Autodesk Fusion 360 part; units mm, degrees
note: some values were not read from the file. Set by a fixed rule: which sketch regions a step uses.
(part 2 of 2)
  spline S320 degree 3 poles (36.333, 6.3383) (36.524, 6.2477) (36.7934, 6.1802) (37.1049, 6.2117) knots 0 0 0 0 1 1 1 1
  spline S321 degree 3 poles (37.1049, 6.2117) (37.645, 6.2677) (38.0601, 6.5293) (38.0394, 7.1055) knots 0 0 0 0 1 1 1 1
  line L71 (38.0394, 7.1055) -> (37.6236, 7.1055)
  spline S322 degree 3 poles (37.6236, 7.1055) (37.6105, 6.9605) (37.5622, 6.7963) (37.4701, 6.7127) knots 0 0 0 0 1 1 1 1
  spline S323 degree 3 poles (37.4701, 6.7127) (37.2798, 6.5385) (36.9031, 6.5393) (36.613, 6.639) knots 0 0 0 0 1 1 1 1
  spline S324 degree 3 poles (36.613, 6.639) (36.3852, 6.7173) (36.3092, 7.0603) (36.399, 7.2368) knots 0 0 0 0 1 1 1 1
  spline S325 degree 3 poles (36.399, 7.2368) (36.4964, 7.427) (36.9998, 7.3472) (37.4548, 7.4539) knots 0 0 0 0 1 1 1 1
  spline S326 degree 3 poles (37.4548, 7.4539) (37.7601, 7.5268) (38.0279, 7.6626) (38.1292, 8.0232) knots 0 0 0 0 1 1 1 1
  spline S327 degree 3 poles (38.1292, 8.0232) (38.196, 8.255) (38.1737, 8.5534) (38.0617, 8.7291) knots 0 0 0 0 1 1 1 1
  spline S328 degree 3 poles (38.0617, 8.7291) (37.797, 9.1389) (37.0911, 9.1757) (36.6506, 8.9002) knots 0 0 0 0 1 1 1 1
  spline S329 degree 3 poles (36.6506, 8.9002) (36.5463, 8.8343) (36.4488, 8.7314) (36.3591, 8.6493) knots 0 0 0 0 1 1 1 1
  spline S330 degree 3 poles (36.3591, 8.6493) (36.3399, 9.0276) (36.0429, 9.1289) (35.6248, 9.0023) knots 0 0 0 0 1 1 1 1
  line L72 (35.6248, 9.0023) -> (35.6271, 8.6678)
  spline S331 degree 3 poles (35.6271, 8.6678) (35.7475, 8.7023) (35.9348, 8.7222) (35.9348, 8.5573) knots 0 0 0 0 1 1 1 1
  spline S332 degree 3 poles (36.4465, 8.3186) (36.5708, 8.5642) (36.9269, 8.7115) (37.2399, 8.7115) knots 0 0 0 0 1 1 1 1
  spline S333 degree 3 poles (37.2399, 8.7115) (37.4655, 8.7115) (37.6619, 8.6079) (37.7003, 8.3301) knots 0 0 0 0 1 1 1 1
  spline S334 degree 3 poles (37.7003, 8.3301) (37.7225, 8.2166) (37.7011, 8.0984) (37.6412, 7.9994) knots 0 0 0 0 1 1 1 1
  spline S335 degree 3 poles (37.6412, 7.9994) (37.5507, 7.859) (37.3404, 7.7961) (36.9921, 7.7639) knots 0 0 0 0 1 1 1 1
  spline S336 degree 3 poles (36.9921, 7.7639) (36.7642, 7.7439) (36.4887, 7.6779) (36.3782, 7.6173) knots 0 0 0 0 1 1 1 1
  spline S337 degree 3 poles (36.3782, 7.6173) (36.3744, 7.8414) (36.366, 8.1629) (36.4458, 8.3179) knots 0 0 0 0 1 1 1 1
  line L73 (36.4458, 8.3179) -> (36.4465, 8.3186)
  line L74 (32.4735, 5.2733) -> (32.0277, 5.2733)
  line L75 (32.0277, 5.2733) -> (32.0277, 9.0138)
  line L76 (32.0277, 9.0138) -> (32.4735, 9.0138)
  line L77 (32.4735, 9.0138) -> (32.4735, 5.2733)
extrude "Extrude3" add sketch "Sketch3" along normal blind 0.0254 separate body contours S0 L0 S1 L1 S2 L2 S3 L3 | S4 S5 S6 S7 S8 S9 S10 S11 | S17 S18 S19 S20 S21 L5 S22 L6 S23 S24 S25 L7 S26 | S27 S28 S29 S30 S31 S32 S33 S34 S35 S36 S37 S38 L8 S39 S40 S41 S42 S43 S44 S45 S46 S47 S48 S49 | S70 S71 L11 S72 S73 L12 S74 S75 S76 S77 S78 S79 S80 L13 S81 S82 L14 S83 L15 S84 S85 S86 S87 S88 | S105 S106 S107 S108 S109 S110 S111 S112 S113 | L23 S118 L24 S119 S120 S121 L25 S122 | S125 S126 L28 S127 L29 S128 S129 S130 | S138 S139 S140 L32 S141 S142 S143 S144 S145 S146 L33 S147 S148 S149 S150 S151 S152 S153 | L35 L36 L37 L38 L39 L40 L41 L42 | S154 S155 S156 S157 S158 S159 S160 S161 S162 S163 S164 S165 S166 | S179 S180 S181 S182 S183 S184 S185 S186 | S195 S196 S197 L43 S198 S199 S200 S201 S202 S203 S204 S205 S206 S207 S208 S209 S210 S211 | S241 S242 S243 S244 S245 L48 | S256 S257 S258 L52 S259 | S271 S272 S273 S274 S275 S276 S277 | S292 S293 S294 S295 | S300 S301 S302 S303 | S313 S314 S315 S316 S317 | S332 S333 S334 S335 S336 S337 makes body 9 at (-34.5529, 8.7319, 1.2) makes body 10 at (-46.775, 8.4751, 1.2) makes body 11 at (-39.8222, -6.911, 1.2) makes body 12 at (-45.931, -5.1825, 1.2) makes body 13 at (-39.0116, -2.8821, 1.2) makes body 14 at (-44.064, 0.5433, 1.2) makes body 15 at (-52.6712, -6.0914, 1.2) makes body 16 at (-37.4749, -8.2903, 1.2) makes body 17 at (-43.7213, 8.8667, 1.2) makes body 18 at (-32.2524, 9.33, 1.2) makes body 19 at (-37.1847, 8.8219, 1.2) makes body 20 at (-30.552, -7.1404, 1.2) makes body 21 at (-44.0732, -8.4989, 1.2) makes body 22 at (-52.7735, 1.0137, 1.2) makes body 23 at (-30.9607, 6.6167, 1.2) makes body 24 at (-48.0874, 5.5522, 1.2) makes body 25 at (-49.5945, -7.1405, 1.2) makes body 26 at (-34.0945, -6.9023, 1.2) makes body 27 at (-41.1326, 9.0477, 1.2) makes body 28 at (-28.8401, 9.9626, 1.2)
